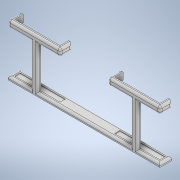
# Autodesk Inventor part: Mount&holder
Saved by Autodesk Inventor 2020 (Build 240168000, 168)
## iProperties
Created: 2020-03-06
Part Number: Mount&holder
Material: Generic
Document SubType Name: Modeling
Designer: Sverrir
Density: 1 g/cm^3
Appearance: Default
Author: Sverrir
Autodesk Inventor part; units mm, degrees
ref_plane "YZ Plane" through (0, 0, 0) normal (1, 0, 0) x (0, 1, 0)
ref_plane "XZ Plane" through (0, 0, 0) normal (0, 1, 0) x (-1, 0, 0)
ref_plane "XY Plane" through (0, 0, 0) normal (0, 0, 1) x (1, 0, 0)
sketch "Sketch2" plane through (0, 0, 0) normal (0, 1, 0) x (-1, 0, 0)
  line L0 (114.05, -25.6474) -> (-114.05, -25.6474)
  line L1 (-114.05, -25.6474) -> (-114.05, -7.6474)
  line L2 (-114.05, -7.6474) -> (114.05, -7.6474)
  line L3 (114.05, -7.6474) -> (114.05, -25.6474)
  line L4 (109.05, -20.6474) -> (40.95, -20.6474) construction
  line L5 (40.95, -20.6474) -> (40.95, -12.6474) construction
  line L6 (40.95, -12.6474) -> (109.05, -12.6474) construction
  line L7 (109.05, -12.6474) -> (109.05, -20.6474) construction
  line L8 (40.95, -20.6474) -> (109.05, -12.6474) construction
  line L9 (109.05, -20.6474) -> (40.95, -12.6474) construction
  line L10 (-40.95, -20.6474) -> (-109.05, -20.6474) construction
  line L11 (-109.05, -20.6474) -> (-109.05, -12.6474) construction
  line L12 (-109.05, -12.6474) -> (-40.95, -12.6474) construction
  line L13 (-40.95, -12.6474) -> (-40.95, -20.6474) construction
  line L14 (-109.05, -20.6474) -> (-40.95, -12.6474) construction
  line L15 (-40.95, -20.6474) -> (-109.05, -12.6474) construction
  line L16 (0, 0) -> (0, -43.252) construction
  point P0 (75, -16.6474)
  point P1 (-75, -16.6474)
  dimension "d6" = 68.1
  dimension "d7" = 8
  dimension "d8" = 68.1
  dimension "d9" = 8
  dimension "d10" = 5
  dimension "d11" = 5
  dimension "d12" = 5
  dimension "d13" = 5
  dimension "d14" = 150
  constraints: 34 end point, 6 parallel, 3 horizontal, 3 perpendicular, 2 midpoint, 1 collinear, 1 vertical, 1 other
  measures "d6" distance of L5.end L6.end
  measures "d7" distance of L4.end L5.end
  measures "d8" distance of L11.end L12.end
  measures "d9" distance of L10.end L11.end
  measures "d10" distance between parallel lines of L1 L11
  measures "d11" distance between parallel lines of L3 L7
  measures "d12" distance between parallel lines of L0 L4
  measures "d13" distance between parallel lines of L2 L6
  measures "d14" distance of point (75, -16.647) point (-75, -16.647)
extrude "Extrusion1" add sketch "Sketch2" against normal blind 5
sketch "Sketch6" plane through (0, 0, 0) normal (0, 1, 0) x (1, 0, 0)
  line L0 (-109.05, 12.6474) -> (-109.05, 20.6474) construction
  line L1 (-109.05, 20.6474) -> (-40.95, 20.6474) construction
  line L2 (-40.95, 20.6474) -> (-40.95, 12.6474) construction
  line L3 (-40.95, 12.6474) -> (-109.05, 12.6474) construction
  line L4 (40.95, 12.6474) -> (40.95, 20.6474) construction
  line L5 (40.95, 20.6474) -> (109.05, 20.6474) construction
  line L6 (109.05, 20.6474) -> (109.05, 12.6474) construction
  line L7 (109.05, 12.6474) -> (40.95, 12.6474) construction
  line L8 (-109.05, 20.6474) -> (-40.95, 20.6474)
  line L9 (-40.95, 20.6474) -> (-40.95, 12.6474)
  line L10 (-40.95, 12.6474) -> (-109.05, 12.6474)
  line L11 (-109.05, 12.6474) -> (-109.05, 20.6474)
  line L12 (40.95, 20.6474) -> (109.05, 20.6474)
  line L13 (109.05, 20.6474) -> (109.05, 12.6474)
  line L14 (109.05, 12.6474) -> (40.95, 12.6474)
  line L15 (40.95, 12.6474) -> (40.95, 20.6474)
  point P0 (0, 0)
  constraints: 16 end point, 4 parallel, 2 horizontal, 2 perpendicular
extrude "Extrusion2" cut sketch "Sketch6" against normal blind 1
sketch "Sketch7" plane through (0, 0, 0) normal (0, 1, 0) x (1, 0, 0)
  line L0 (-109.05, 12.6474) -> (-109.05, 20.6474) projected
  line L1 (-40.95, 12.6474) -> (-109.05, 12.6474) projected
  line L2 (-40.95, 20.6474) -> (-40.95, 12.6474) projected
  line L3 (-109.05, 20.6474) -> (-40.95, 20.6474) projected
  line L4 (40.95, 12.6474) -> (40.95, 20.6474) projected
  line L5 (109.05, 12.6474) -> (40.95, 12.6474) projected
  line L6 (109.05, 20.6474) -> (109.05, 12.6474) projected
  line L7 (40.95, 20.6474) -> (109.05, 20.6474) projected
  line L8 (-80, 7.6474) -> (-70, 7.6474)
  line L9 (-70, 7.6474) -> (-70, 12.6474)
  line L10 (-70, 12.6474) -> (-80, 12.6474)
  line L11 (-80, 12.6474) -> (-80, 7.6474)
  line L12 (70, 7.6474) -> (80, 7.6474)
  line L13 (80, 7.6474) -> (80, 12.6474)
  line L14 (80, 12.6474) -> (70, 12.6474)
  line L15 (70, 12.6474) -> (70, 7.6474)
  line L16 (109.05, 12.6474) -> (40.95, 12.6474) projected
  line L17 (40.95, 12.6474) -> (40.95, 20.6474) projected
  line L18 (40.95, 20.6474) -> (109.05, 20.6474) projected
  line L19 (109.05, 20.6474) -> (109.05, 12.6474) projected
  line L20 (-40.95, 12.6474) -> (-109.05, 12.6474) projected
  line L21 (-109.05, 12.6474) -> (-109.05, 20.6474) projected
  line L22 (-109.05, 20.6474) -> (-40.95, 20.6474) projected
  line L23 (-40.95, 20.6474) -> (-40.95, 12.6474) projected
  line L24 (114.05, 25.6474) -> (-114.05, 25.6474) projected
  line L25 (-114.05, 25.6474) -> (-114.05, 7.6474) projected
  line L26 (-114.05, 7.6474) -> (114.05, 7.6474) projected
  line L27 (114.05, 7.6474) -> (114.05, 25.6474) projected
  line L28 (-114.05, 7.6474) -> (114.05, 7.6474) projected
  line L29 (-40.95, 12.6474) -> (-109.05, 12.6474) projected
  point P0 (0, 0)
  point P1 (-75, 12.6474)
  point P2 (75, 12.6474)
  dimension "d17" = 10
  dimension "d19" = 10
  constraints: 16 end point, 4 midpoint, 4 parallel, 2 collinear, 2 horizontal, 2 perpendicular, 1 point on line
  measures "d17" distance of L8.start L8.end
  measures "d19" distance of L12.start L12.end
extrude "Extrusion3" add sketch "Sketch7" along normal blind 62.9125 contours L1 L9 L8 L11 | L15 L5 L13 L12
sketch "Sketch8" plane through (0, 62.9125, 0) normal (0, 1, 0) x (1, 0, 0)
  line L0 (40.95, 12.6474) -> (40.95, 20.6474) projected
  line L1 (109.05, 12.6474) -> (40.95, 12.6474) projected
  line L2 (109.05, 20.6474) -> (109.05, 12.6474) projected
  line L3 (40.95, 20.6474) -> (109.05, 20.6474) projected
  line L4 (-109.05, 12.6474) -> (-109.05, 20.6474) projected
  line L5 (-40.95, 12.6474) -> (-109.05, 12.6474) projected
  line L6 (-40.95, 20.6474) -> (-40.95, 12.6474) projected
  line L7 (-109.05, 20.6474) -> (-40.95, 20.6474) projected
  line L8 (-114.05, 7.6474) -> (-114.05, 25.6474) projected
  line L9 (-114.05, 25.6474) -> (114.05, 25.6474) projected
  line L10 (-114.05, 7.6474) -> (-35.95, 7.6474)
  line L11 (-35.95, 7.6474) -> (-35.95, 25.6474)
  line L12 (-114.05, 25.6474) -> (-114.05, 7.6474)
  line L13 (-40.95, 25.6474) -> (-40.95, 12.6474)
  line L14 (-40.95, 12.6474) -> (-109.05, 12.6474) projected
  line L15 (-109.05, 12.6474) -> (-109.05, 25.6474)
  line L16 (-35.95, 25.6474) -> (-40.95, 25.6474)
  line L17 (-109.05, 25.6474) -> (-114.05, 25.6474)
  line L18 (114.05, 7.6474) -> (114.05, 25.6474) projected
  line L19 (114.05, 7.6474) -> (35.95, 7.6474)
  line L20 (35.95, 7.6474) -> (35.95, 25.6474)
  line L21 (114.05, 25.6474) -> (114.05, 7.6474)
  line L22 (109.05, 25.6474) -> (109.05, 12.6474)
  line L23 (40.95, 12.6474) -> (40.95, 20.6474) projected
  line L24 (40.95, 12.6474) -> (40.95, 25.6474)
  line L25 (35.95, 25.6474) -> (40.95, 25.6474)
  line L26 (109.05, 25.6474) -> (114.05, 25.6474)
  point P0 (0, 0)
  dimension "d22" = 5
  dimension "d25" = 5
  constraints: 28 end point, 6 parallel, 4 perpendicular, 2 collinear, 2 horizontal, 2 point on line
  measures "d22" distance between parallel lines of L6 L11
  measures "d25" distance between parallel lines of L0 L20
extrude "Extrusion4" add sketch "Sketch8" along normal blind 10.525 contours L1 L2 L22 L9 L18 L19 L20 L24 L0 | L5 L6 L13 L9 L11 L10 L8 L15 L4
fillet "Fillet1" radius 3.175 32 edges at (0, 0, -25.6474) (-114.05, 73.4375, -16.6474) (-114.05, 62.9125, -16.6474) (-35.95, 73.4375, -16.6474) (-35.95, 62.9125, -16.6474) (-35.95, 68.175, -25.6474) (-35.95, 68.175, -7.6474) (-114.05, 68.175, -25.6474) (-114.05, 68.175, -7.6474) (-75, 73.4375, -7.6474) (-52.975, 62.9125, -7.6474) (-97.025, 62.9125, -7.6474) (-80, 31.4562, -7.6474) (-70, 31.4562, -7.6474) (35.95, 62.9125, -16.6474) (35.95, 73.4375, -16.6474) (35.95, 68.175, -7.6474) (52.975, 62.9125, -7.6474) (75, 73.4375, -7.6474) (70, 31.4562, -7.6474) (80, 31.4562, -7.6474) (97.025, 62.9125, -7.6474) (114.05, 68.175, -7.6474) (0, 0, -7.6474) (-97.025, 0, -7.6474) (97.025, 0, -7.6474) (114.05, 73.4375, -16.6474) (114.05, 62.9125, -16.6474) (114.05, 68.175, -25.6474) (35.95, 68.175, -25.6474) (-114.05, 0, -16.6474) (114.05, 0, -16.6474)
equation "\"d10\" = d12"
equation "\"d11\" = d12"
equation "\"d19\" = d17"
equation "\"d25\" = d22"
body "Solid1"
